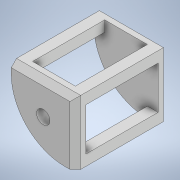
# Autodesk Inventor part: 16-1
Saved by Autodesk Inventor 2022 (Build 260153000, 153)
## iProperties
Created: 2021-09-25
Part Number: 16-1
Material: 일반
Document SubType Name: Modeling
Designer: 서울공업고등학교
Density: 1 g/cm^3
Appearance: 기본값
Author: 서울공업고등학교
Autodesk Inventor part; units mm, degrees
ref_plane "YZ Plane" through (0, 0, 0) normal (1, 0, 0) x (0, 1, 0)
ref_plane "XZ Plane" through (0, 0, 0) normal (0, 1, 0) x (-1, 0, 0)
sketch "스케치1" plane through (0, 0, 0) normal (0, 0, 1) x (1, 0, 0)
  line L0 (0, 0) -> (24, 0)
  line L1 (24, 0) -> (24, -24)
  line L2 (24, -24) -> (0, -24)
  line L3 (0, -24) -> (0, 0)
  circle A0 centre (12, -12) radius 2.5
  dimension "d0" = 24
  dimension "d1" = 24
  dimension "d2" = 5
  dimension "d3" = 12
  dimension "d4" = 12
  constraints: 8 end point, 2 parallel, 1 centre point, 1 horizontal, 1 perpendicular
  measures "d0" distance of L1.end L2.end
  measures "d1" distance of L0.end L1.end
  measures "d2" diameter of A0
  measures "d3" distance from line of A0.centre L0
  measures "d4" distance from line of A0.centre L3
extrude "돌출1" add sketch "스케치1" along normal mid plane 35
fillet "모깎기1" radius 20 1 edges at (0, -24, 0)
chamfer "모따기1" distance 2 angle 45 4 edges at (12, 0, 17.5) (12, 0, -17.5) (24, -12, 17.5) (24, -12, -17.5)
ref_plane "작업 평면1" through (0, 0, 0) normal (0, 0, 1) x (1, 0, 0)
sketch "스케치2" plane through (0, 0, 0) normal (0, 0, 1) x (1, 0, 0)
  line L0 (24, -24) -> (24, 0) projected
  line L1 (24, 0) -> (20, 0)
  line L2 (20, 0) -> (20, -4)
  line L3 (20, -4) -> (24, -4)
  line L4 (24, -4) -> (24, 0)
  line L5 (0, 0) -> (0, -2) projected
  line L6 (0, 0) -> (4, 0)
  line L7 (4, 0) -> (4, -4)
  line L8 (4, -4) -> (0, -4)
  line L9 (0, -4) -> (0, 0)
  line L10 (22, -24) -> (24, -24) projected
  line L11 (24, -24) -> (20, -24)
  line L12 (20, -24) -> (20, -20)
  line L13 (20, -20) -> (24, -20)
  line L14 (24, -20) -> (24, -24)
  line L15 (22, -2) -> (24, 0) projected
  line L16 (24, 0) -> (0, 0)
  line L17 (0, 0) -> (0, -24)
  line L18 (0, -24) -> (24, -24)
  line L19 (24, -24) -> (24, 0)
  dimension "d11" = 4
  dimension "d12" = 4
  dimension "d13" = 4
  dimension "d14" = 4
  dimension "d15" = 4
  constraints: 32 end point, 8 parallel, 4 horizontal, 4 perpendicular, 1 point on line
  measures "d11" distance of L3.end L2.end
  measures "d12" distance of L2.end L1.end
  measures "d13" distance of L7.end L8.end
  measures "d14" distance of L12.end L13.end
  measures "d15" distance of L11.end L12.end
extrude "돌출2" cut sketch "스케치2" along normal mid plane 27 contours L13 L12 L18 L17 L8 L7 L16 L2 L3 L0
